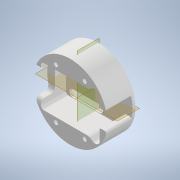
# Autodesk Inventor part: Manatee_bottom_v0
Saved by Autodesk Inventor 2022 (Build 260153000, 153)
## iProperties
Created: 2022-03-17
Part Number: Manatee_bottom_v0
Material: Generic
Document SubType Name: Modeling
Designer: Prakash Lab
Density: 1 g/cm^3
Appearance: Default
Author: Prakash Lab
Autodesk Inventor part; units mm, degrees
ref_plane "YZ Plane" through (0, 0, 0) normal (1, 0, 0) x (0, 1, 0)
ref_plane "XZ Plane" through (0, 0, 0) normal (0, 1, 0) x (-1, 0, 0)
ref_plane "XY Plane" through (0, 0, 0) normal (0, 0, 1) x (1, 0, 0)
sketch "Sketch6" plane through (0, 0, 0) normal (0, 0, 1) x (1, 0, 0)
  circle A0 centre (0, 0) radius 26
  dimension "d33" = 52
  constraints: 1 centre point, 1 coincident
  measures "d33" diameter of A0
extrude "Extrusion5" add sketch "Sketch6" along normal blind 2
sketch "Sketch7" plane through (0, 0, 2) normal (0, 0, 1) x (1, 0, 0)
  line L0 (-20.5, 14.25) -> (20.5, 14.25)
  line L1 (20.5, 14.25) -> (20.5, -14.25)
  line L2 (20.5, -14.25) -> (-20.5, -14.25)
  line L3 (-20.5, -14.25) -> (-20.5, 14.25)
  line L4 (-20.5, 14.25) -> (20.5, -14.25) construction
  line L5 (20.5, 14.25) -> (-20.5, -14.25) construction
  circle A0 centre (0, 0) radius 26 projected
  point P0 (20.5, -15.9922)
  point P1 (-20.5, -15.9922)
  point P2 (-20.5, 15.9922)
  point P3 (20.5, 15.9922)
  dimension "d36" = 41
  dimension "d37" = 28.5
  constraints: 12 end point, 2 midpoint, 2 parallel, 1 coincident, 1 horizontal, 1 perpendicular
  measures "d36" distance of L1.end L2.end
  measures "d37" distance of L0.end L1.end
extrude "Extrusion6" add sketch "Sketch7" along normal blind 17.5
fillet "Fillet2" radius 2 4 edges at (-20.5, 14.25, 10.75) (-20.5, -14.25, 10.75) (20.5, -14.25, 10.75) (20.5, 14.25, 10.75)
sketch "Sketch8" plane through (0, 0, 19.5) normal (0, 0, 1) x (1, 0, 0)
  circle A0 centre (0, 0) radius 26 projected
  line L0 (-18.5, 14.25) -> (18.5, 14.25) projected
  arc A1 (20.5, 12.25) -> (18.5, 14.25) centre (18.5, 12.25) ccw projected
  line L1 (20.5, 12.25) -> (20.5, -12.25) projected
  arc A2 (18.5, -14.25) -> (20.5, -12.25) centre (18.5, -12.25) ccw projected
  line L2 (18.5, -14.25) -> (-18.5, -14.25) projected
  arc A3 (-20.5, -12.25) -> (-18.5, -14.25) centre (-18.5, -12.25) ccw projected
  line L3 (-20.5, -12.25) -> (-20.5, 12.25) projected
  arc A4 (-18.5, 14.25) -> (-20.5, 12.25) centre (-18.5, 12.25) ccw projected
  line L4 (26.8629, 6.4938) -> (20.5, 6.4938)
  line L5 (20.5, 6.4938) -> (20.5, -5.4938)
  line L6 (20.5, -5.4938) -> (26.8629, -5.4938)
  line L7 (26.8629, -5.4938) -> (26.8629, 6.4938)
  line L8 (26.8629, 6.4938) -> (20.5, -5.4938) construction
  line L9 (20.5, 6.4938) -> (26.8629, -5.4938) construction
  point P0 (23.6815, 0.5)
  point P1 (25.4129, -5.4938)
  point P2 (25.176, 6.4938)
  point P3 (20.5, 6.4938)
  constraints: 12 end point, 2 midpoint, 2 parallel, 1 horizontal, 1 perpendicular, 1 point on line
extrude "Extrusion7" cut sketch "Sketch8" against normal up to surface (17.5 mm away) contours A0 L6 L1 L4
sketch "Sketch9" plane through (0, 0, 0) normal (0, 0, -1) x (-1, 0, 0)
  arc A0 (-25.4129, -5.4938) -> (-25.176, 6.4938) centre (0, 0) ccw projected
  line L0 (-25.4129, -5.4938) -> (-20.5, -5.4938) projected
  line L1 (-20.5, 12.25) -> (-20.5, 6.4938) projected
  arc A1 (-20.5, -12.25) -> (-18.5, -14.25) centre (-18.5, -12.25) ccw projected
  line L2 (-18.5, -14.25) -> (18.5, -14.25) projected
  arc A2 (18.5, -14.25) -> (20.5, -12.25) centre (18.5, -12.25) ccw projected
  line L3 (20.5, -12.25) -> (20.5, 12.25) projected
  arc A3 (20.5, 12.25) -> (18.5, 14.25) centre (18.5, 12.25) ccw projected
  line L4 (18.5, 14.25) -> (-18.5, 14.25) projected
  line L5 (10, -17.5) -> (-10, -17.5)
  line L6 (-10, -17.5) -> (-10, 17.5)
  line L7 (-10, 17.5) -> (10, 17.5)
  line L8 (10, 17.5) -> (10, -17.5)
  line L9 (10, -17.5) -> (-10, 17.5) construction
  line L10 (-10, -17.5) -> (10, 17.5) construction
  line L11 (-20.5, -5.4938) -> (-20.5, -12.25) projected
  arc A4 (-18.5, 14.25) -> (-20.5, 12.25) centre (-18.5, 12.25) ccw projected
  line L12 (-20.5, 6.4938) -> (-25.176, 6.4938) projected
  dimension "d44" = 20
  dimension "d45" = 35
  constraints: 12 end point, 2 midpoint, 2 parallel, 1 horizontal, 1 perpendicular
  measures "d44" distance of L6.end L7.end
  measures "d45" distance of L5.end L6.end
hole "Hole2" at (10, 17.5, 0) at (-10, 17.5, 0) at (-10, -17.5, 0) at (10, -17.5, 0) direction (0, 0, 1) diameter 2.8 end through all start extended yes counterbore diameter 6.5 counterbore depth 3
ref_plane "Work Plane4" through (-18.5, 0, 2) normal (0, 1, 0) x (1, 0, 0)
ref_plane "Work Plane5" through (0, -12.25, 2) normal (-1, 0, 0) x (0, 0, 1)
fillet "Fillet4" radius 1 4 edges at (25.4129, -5.4938, 10.75) (25.176, 6.4938, 10.75) (20.5, -5.4938, 10.75) (20.5, 6.4938, 10.75)
sketch "Sketch11" plane through (0, -12.25, 2) normal (-1, 0, 0) x (0, 0, 1)
  line L0 (-5.9, 12.25) -> (21.4, 12.25) projected
  line L1 (0, 20.0436) -> (0, 5.4964) projected
  line L2 (17.5, 5.4964) -> (0, 5.4964) projected
  line L3 (17.5, 20.0436) -> (17.5, 5.4964) projected
  line L4 (0, 20.0436) -> (17.5, 20.0436) projected
  line L5 (-2, -13.75) -> (-2, 38.25) projected
  line L6 (7.5, 3.25) -> (17.5, 3.25)
  line L7 (17.5, 3.25) -> (17.5, 21.25)
  line L8 (17.5, 21.25) -> (7.5, 21.25)
  line L9 (7.5, 21.25) -> (7.5, 3.25)
  line L10 (7.5, 3.25) -> (17.5, 21.25) construction
  line L11 (17.5, 3.25) -> (7.5, 21.25) construction
  point P0 (-2, 12.25)
  point P1 (12.5, 12.25)
  dimension "d59" = 18
  dimension "d60" = 10
  constraints: 12 end point, 2 midpoint, 2 parallel, 2 point on line, 1 horizontal, 1 perpendicular
  measures "d59" distance of L6.end L7.end
  measures "d60" distance between parallel lines of L9 L7
extrude "Extrusion8" cut sketch "Sketch11" along normal through all contours L9 L4 L3 L0 | L0 L3 L2 L9 | L9 L8 L7 L4 | L2 L7 L6 L9
fillet "Fillet5" radius 3 4 edges at (-22.4463, 9, 19.5) (-22.4463, 9, 9.5) (-22.4463, -9, 19.5) (-22.4463, -9, 9.5)
sketch "Sketch12" plane through (0, 0, 0) normal (0, 0, -1) x (-1, 0, 0)
  line L0 (15.5975, 10.9803) -> (15.5975, 11.6153) projected
  line L1 (-2.5665, 11.2343) -> (-2.8205, 10.9803) projected
  line L2 (-2.8275, -11.3847) -> (-2.8275, -12.0197) projected
  line L3 (15.6075, -12.0197) -> (15.6075, -11.3847) projected
  line L4 (15.5975, 10.9803) -> (-2.8205, 10.9803) construction
  line L5 (15.5975, 13.5462) -> (-2.8205, 13.5462)
  line L6 (-2.8205, 8.4145) -> (15.5975, 8.4145)
  arc A0 (15.5975, 8.4145) -> (15.5975, 13.5462) centre (15.5975, 10.9803) ccw
  arc A1 (-2.8205, 13.5462) -> (-2.8205, 8.4145) centre (-2.8205, 10.9803) ccw
  line L7 (15.6075, -11.3847) -> (-2.8275, -11.3847) construction
  line L8 (15.6075, -8.8258) -> (-2.8275, -8.8258)
  line L9 (-2.8275, -13.9435) -> (15.6075, -13.9435)
  arc A2 (15.6075, -13.9435) -> (15.6075, -8.8258) centre (15.6075, -11.3847) ccw
  arc A3 (-2.8275, -8.8258) -> (-2.8275, -13.9435) centre (-2.8275, -11.3847) ccw
  point P0 (0, 0)
  point P1 (-2.4395, 11.3613)
  point P2 (6.3885, 10.9803)
  point P3 (6.39, -11.3847)
  constraints: 16 end point, 8 point on circle, 8 tangent, 4 centre point, 3 parallel, 2 midpoint, 1 horizontal, 1 other
extrude "Extrusion9" cut sketch "Sketch12" against normal blind 25.4
sketch "Sketch13" plane through (0, 0, 19.5) normal (0, 0, 1) x (1, 0, 0)
  circle A0 centre (0.0002, -0.0021) radius 25.9979
  line L0 (18.5, -14.25) -> (-18.5, -14.25) projected
  arc A1 (18.5, -14.25) -> (20.5, -12.25) centre (18.5, -12.25) ccw projected
  line L1 (20.5, -6.4938) -> (20.5, -12.25) projected
  line L2 (-18.5, 14.25) -> (18.5, 14.25) projected
  arc A2 (20.5, 12.25) -> (18.5, 14.25) centre (18.5, 12.25) ccw projected
  line L3 (20.5, 12.25) -> (20.5, 7.4938) projected
  arc A3 (20.5, 12.25) -> (18.5, 14.25) centre (18.5, 12.25) ccw projected
  arc A4 (20.5, 12.25) -> (14.25, 14.25) centre (17.375, 13.25) ccw
  line L4 (10, -14.25) -> (18.5, -14.25) projected
  line L5 (20.5, -12.25) -> (20.5, -6.4938) projected
  arc A5 (14.25, -14.25) -> (20.5, -12.25) centre (17.375, -13.25) ccw
  point P0 (0, 0)
  constraints: 4 point on circle, 3 centre point, 2 midpoint, 1 point on line, 2 other
extrude "Extrusion10" cut sketch "Sketch13" against normal up to surface (17.5 mm away) contours A1 A5 L0 | A4 A2 L2
fillet "Fillet6" radius 5 2 edges at (14.25, -14.25, 10.75) (14.25, 14.25, 10.75)
body "Solid2"
